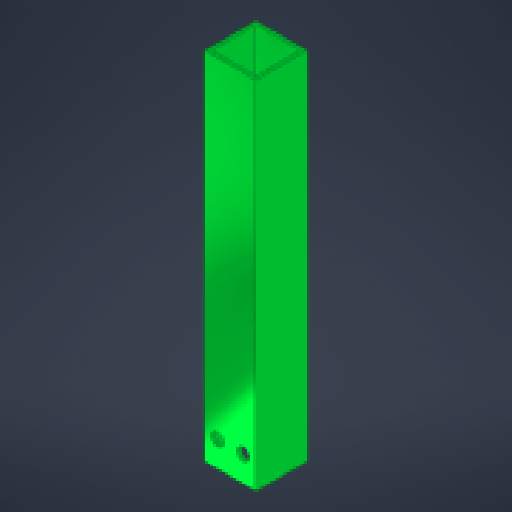
# Autodesk Inventor part: 1
Saved by Autodesk Inventor 2024 (Build 280153000, 153)
## iProperties
Created: 2023-04-17
Part Number: 1
Material: Алюминий 6061
Document SubType Name: Modeling
Designer: user
Density: 2.7 g/cm^3
Appearance: Алюминий — плоский
Mass: 41.3402 g
Surface Area: 207.312 cm^2
Volume: 15.3112 cm^3
Author: user
Autodesk Inventor part; units mm, degrees
ref_plane "YZ Plane" through (0, 0, 0) normal (1, 0, 0) x (0, 1, 0)
ref_plane "XZ Plane" through (0, 0, 0) normal (0, 1, 0) x (-1, 0, 0)
ref_plane "XY Plane" through (0, 0, 0) normal (0, 0, 1) x (1, 0, 0)
sketch "Эскиз1" plane through (0, 0, 0) normal (0, 0, 1) x (1, 0, 0)
  line L0 (0, 0) -> (20, 0)
  line L1 (20, 0) -> (20, 20)
  line L2 (20, 20) -> (0, 20)
  line L3 (0, 20) -> (0, 0)
  line L4 (1.5, 1.5) -> (18.5, 1.5)
  line L5 (18.5, 1.5) -> (18.5, 18.5)
  line L6 (18.5, 18.5) -> (1.5, 18.5)
  line L7 (1.5, 18.5) -> (1.5, 1.5)
  point P0 (10, 18.5)
  point P1 (10, 20)
  point P2 (18.5, 10)
  point P3 (20, 10)
  dimension "d0" = 20
  dimension "d1" = 1.5
  constraints: 16 end point, 4 midpoint, 4 parallel, 4 perpendicular, 2 horizontal, 1 horizontal alignment, 1 vertical alignment
  measures "d0" distance of L1.end L2.end
  measures "d1" horizontal distance of L1.end L5.end
extrude "Выдавливание1" add sketch "Эскиз1" along normal blind 139
sketch "Эскиз2" plane through (0, 20, 0) normal (0, 1, 0) x (1, 0, 0)
  circle A0 centre (5, -10) radius 2.5
  circle A1 centre (15, -10) radius 2.5
  line L0 (5, -10) -> (15, -10) construction
  line L1 (20, 0) -> (0, 0) construction
  point P0 (10, -10)
  point P1 (10, 0)
  point P2 (10, 0)
  dimension "d4" = 10
  dimension "d5" = 5
  dimension "d6" = 10
  constraints: 3 midpoint, 2 centre point, 2 end point, 1 equal radius, 1 horizontal, 1 vertical alignment
  measures "d4" vertical distance of point (10, 0) L0.start
  measures "d5" diameter of A1
  measures "d6" distance of L0.start L0.end
extrude "Выдавливание2" cut sketch "Эскиз2" against normal through all
